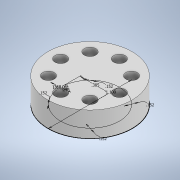
# Autodesk Inventor part: Collector rotation xrail to turntable adapter
Saved by Autodesk Inventor 2020 (Build 240168000, 168)
## iProperties
Created: 2019-12-31
Part Number: Collector rotation xrail to turntable adapter
Material: Generic
Document SubType Name: Modeling
Designer: FTC8863
Density: 1 g/cm^3
Appearance: Default
Author: FTC8863
Autodesk Inventor part; units mm, degrees
ref_plane "YZ Plane" through (0, 0, 0) normal (1, 0, 0) x (0, 1, 0)
ref_plane "XZ Plane" through (0, 0, 0) normal (0, 1, 0) x (-1, 0, 0)
ref_plane "XY Plane" through (0, 0, 0) normal (0, 0, 1) x (1, 0, 0)
sketch "Sketch1" plane through (0, 0, 0) normal (0, 1, 0) x (-1, 0, 0)
  circle A0 centre (9.779, 0) radius 1.9304 construction
  circle A1 centre (6.9148, 6.9148) radius 1.9304 construction
  circle A2 centre (0, 9.779) radius 1.9304 construction
  circle A3 centre (-6.9148, 6.9148) radius 1.9304 construction
  circle A4 centre (-9.779, 0) radius 1.9304 construction
  circle A5 centre (-6.9148, -6.9148) radius 1.9304 construction
  circle A6 centre (0, -9.779) radius 1.9304 construction
  circle A7 centre (6.9148, -6.9148) radius 1.9304 construction
  circle A8 centre (9.779, 0) radius 3.1242 construction
  circle A9 centre (0, 9.779) radius 3.1242 construction
  circle A10 centre (-9.779, 0) radius 3.1242 construction
  circle A11 centre (0, -9.779) radius 3.1242 construction
  circle A12 centre (0, 0) radius 13.97
  circle A13 centre (6.9148, -6.9148) radius 1.9304
  circle A14 centre (6.9148, 6.9148) radius 1.9304
  circle A15 centre (-6.9148, 6.9148) radius 1.9304
  circle A16 centre (-6.9148, -6.9148) radius 1.9304
  dimension "d0" = 3.8608
  dimension "d1" = 9.779
  dimension "d4" = 360
  dimension "d6" = 6.2484
  dimension "d9" = 360
  dimension "d11" = 27.94
  dimension "d12" = 3.8608
  dimension "d13" = 3.8608
  dimension "d14" = 3.8608
  dimension "d15" = 3.8608
  constraints: 17 centre point, 6 coincident, 26 other
  measures "d0" diameter of A0
  measures "d1" distance of point (0, 0) A0.centre
  measures "d6" diameter of A8
  measures "d11" diameter of A12
  measures "d12" diameter of A13
  measures "d13" diameter of A14
  measures "d14" diameter of A15
  measures "d15" diameter of A16
extrude "Extrusion1" add sketch "Sketch1" along normal blind 8.1788
hole "Hole1" at (0, 0, 9.779) at (9.779, 0, 0) at (0, 0, -9.779) at (-9.779, 0, 0) direction (0, 1, 0) diameter 3.8608 end through all counterbore diameter 6.2484 counterbore depth 4.953
body "Solid1"
